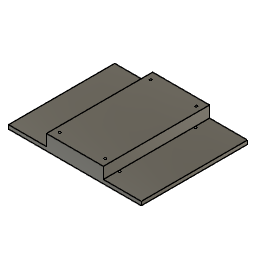
Platform_Riser_V2 (Autodesk Fusion 360 design; units mm, degrees)
part number: 2025-10-16-22-08-15-071
Autodesk Fusion 360 part; units mm, degrees
sketch "Sketch1" plane through (0, 0, 0) normal (0, 0, 1) x (1, 0, 0)
  line L0 (0, 0) -> (175, 0)
  line L1 (175, 0) -> (175, 140)
  line L2 (175, 140) -> (0, 140)
  line L3 (0, 140) -> (0, 0)
  line L4 (50, 140) -> (50, 0)
  line L5 (125, 140) -> (125, 0)
  circle A0 centre (57.5, 10) radius 1.5
  circle A1 centre (117.5, 10) radius 1.5
  line L6 (87.5, 0) -> (87.5, 140) construction
  circle A2 centre (57.5, 130) radius 1.5
  circle A3 centre (117.5, 130) radius 1.5
  line L7 (57.5, 130) -> (57.5, 100) construction
  circle A4 centre (57.5, 107) radius 1.5
  line L8 (117.5, 130) -> (117.5, 100) construction
  circle A5 centre (117.5, 107) radius 1.5
  circle A6 centre (48.5, 120) radius 1.5
  line L9 (0, 70) -> (175, 70) construction
  circle A7 centre (48.5, 20) radius 1.5
  circle A8 centre (126.5, 120) radius 1.5
  circle A9 centre (126.5, 20) radius 1.5
  dimension "d1" = 140
  dimension "d2" = 175
  dimension "d3" = 50
  dimension "d4" = 50
  dimension "d5" = 3
  dimension "d6" = 10
  dimension "d7" = 3
  dimension "d10" = 60
  dimension "d11" = 3
  dimension "d12" = 3
  dimension "d13" = 60
  dimension "d14" = 10
  dimension "d23" = 3
  dimension "d24" = 23
  dimension "d25" = 3
  dimension "d26" = 23
  dimension "d27" = 3
  dimension "d28" = 3
  dimension "d29" = 100
  dimension "d30" = 3
  dimension "d31" = 3
  dimension "d32" = 100
  constraint horizontal L0
  constraint vertical L1
  constraint horizontal L2
  constraint vertical L3
  constraint coincident L0.start L3.end
  constraint coincident L2 L4.start
  constraint coincident L0 L4.end
  constraint perpendicular L0 L4
  constraint coincident L2 L5.start
  constraint coincident L0 L5.end
  constraint perpendicular L0 L5
  constraint midpoint L0 L6.start
  constraint midpoint L2 L6.end
  constraint symmetric A0.centre A1.centre L6
  constraint symmetric L6 A2.centre A3.centre
  constraint coincident A2.centre L7.start
  constraint vertical L7
  constraint coincident L7 A4.centre
  constraint coincident A3.centre L8.start
  constraint vertical L8
  constraint coincident L8 A5.centre
  constraint tangent L4 A6
  constraint midpoint L3 L9.start
  constraint midpoint L1 L9.end
  constraint tangent L4 A7
  constraint symmetric A6.centre L9 A7.centre
  constraint tangent L5 A8
  constraint tangent L5 A9
  constraint symmetric L9 A8.centre A9.centre
  measures "d1" distance of L0.start L2.end
  measures "d2" distance of L0.start L0.end
  measures "d3" distance of L3 L4
  measures "d4" distance of L1 L5
  measures "d5" diameter of A0
  measures "d6" distance of L0 A0.centre
  measures "d7" diameter of A1
  measures "d10" distance of A0.centre A1.centre
  measures "d11" diameter of A2
  measures "d12" diameter of A3
  measures "d13" distance of A2.centre A3.centre
  measures "d14" distance of L2 A2.centre
  measures "d23" diameter of A4
  measures "d24" distance of A2.centre A4.centre
  measures "d25" diameter of A5
  measures "d26" distance of A3.centre A5.centre
  measures "d27" diameter of A6
  measures "d28" diameter of A7
  measures "d29" distance of A6.centre A7.centre
  measures "d30" diameter of A8
  measures "d31" diameter of A9
  measures "d32" distance of A8.centre A9.centre
extrude "Extrude1" add sketch "Sketch1" along normal blind 20 contours L0 L2 L4 L5
extrude "Extrude3" add sketch "Sketch1" along normal blind 5 contours L0 L2 L3 L4 | L0 L1 L2 L5
extrude "Extrude4" add sketch "Sketch1" along normal blind 15 contours A0 | A1
extrude "Extrude5" add sketch "Sketch1" along normal blind 10 from surface at 5 contours A2 | A3
extrude "Extrude6" add sketch "Sketch1" along normal blind 15 from surface at 5 contours A4 | A5
